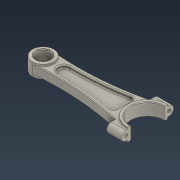
# Autodesk Inventor part: Korbowód
Saved by Autodesk Inventor 2022 (Build 260153000, 153)
## iProperties
Created: 2023-05-22
Part Number: Korbowód
Material: Generic
Document SubType Name: Modeling
Designer: wikto
Density: 1 g/cm^3
Appearance: Steel - Cast
Author: wikto
Autodesk Inventor part; units mm, degrees
ref_plane "YZ Plane" through (0, 0, 0) normal (1, 0, 0) x (0, 1, 0)
ref_plane "XZ Plane" through (0, 0, 0) normal (0, 1, 0) x (-1, 0, 0)
ref_plane "XY Plane" through (0, 0, 0) normal (0, 0, 1) x (1, 0, 0)
sketch "Sketch1" plane through (0, 0, 0) normal (0, 1, 0) x (-1, 0, 0)
  circle A0 centre (49, 0) radius 11
  arc A1 (-121, -27.5) -> (-121, 27.5) centre (-121, 0) ccw
  circle A2 centre (49, 0) radius 12.5
  circle A3 centre (49, 0) radius 17.5
  arc A4 (-121, -32.5) -> (-121, 32.5) centre (-121, 0) ccw
  line L0 (-121, -32.5) -> (-121, -42.5)
  line L1 (-121, -42.5) -> (-96, -42.5)
  line L2 (-121, 32.5) -> (-121, 42.5)
  line L3 (-121, 42.5) -> (-96, 42.5)
  line L4 (-96, -42.5) -> (-96, -27.5)
  line L5 (-96, 42.5) -> (-96, 27.5)
  arc A5 (49, -17.5) -> (-96, -27.5) centre (7.0545, -465.5408) ccw
  arc A6 (-96, 27.5) -> (49, 17.5) centre (7.0545, 465.5408) ccw
  line L6 (-121, -32.5) -> (-121, -27.5)
  line L7 (-121, 32.5) -> (-121, 27.5)
  point P0 (0, 0)
  point P1 (45.8719, 17.2182)
  point P2 (45.8719, -17.2182)
  dimension "d0" = 170
  dimension "d1" = 22
  dimension "d2" = 55
  dimension "d3" = 121
  dimension "d4" = 25
  dimension "d5" = 35
  dimension "d7" = 65
  dimension "d8" = 25
  dimension "d9" = 10
  dimension "d10" = 15
  dimension "d11" = 450
  constraints: 16 end point, 10 point on circle, 7 centre point, 6 vertical, 6 vertical alignment, 3 coincident, 3 equal length, 2 horizontal alignment, 2 perpendicular, 2 point on line, 1 equal radius
  measures "d0" distance of A1.centre A0.centre
  measures "d1" diameter of A0
  measures "d2" diameter of A1
  measures "d3" distance of A1.centre point (0, 0)
  measures "d4" diameter of A2
  measures "d5" diameter of A3
  measures "d7" diameter of A4
  measures "d8" distance of L0.end L1.end
  measures "d9" distance of L0.start L0.end
  measures "d10" distance of L1.end L4.end
  measures "d11" radius of A6
extrude "Extrusion1" add sketch "Sketch1" along normal mid plane 21 contours A1 L7 A4 L6 | A3 A6 A5
extrude "Extrusion2" add sketch "Sketch1" along normal mid plane 15 contours A4 L2 L3 L5 A6 A3 A5 L4 L1 L0
extrude "Extrusion3" add sketch "Sketch1" along normal mid plane 23 contours A2
sketch "Sketch2" plane through (0, 7.5, 0) normal (0, 1, 0) x (1, 0, 0)
  arc A0 (-45.8719, 17.2182) -> (96, 27.5) centre (-7.0545, 465.5408) ccw projected
  arc A1 (96, -27.5) -> (-45.8719, -17.2182) centre (-7.0545, -465.5408) ccw projected
  arc A2 (-14.836, 9.6072) -> (77.0775, 17.3692) centre (-7.0545, 465.5408) ccw
  arc A3 (77.0775, -17.3692) -> (-14.836, -9.6072) centre (-7.0545, -465.5408) ccw
  line L0 (83, 12.455) -> (83, -12.455)
  arc A4 (83, 12.455) -> (77.0775, 17.3692) centre (78, 12.455) ccw
  arc A5 (77.0775, -17.3692) -> (83, -12.455) centre (78, -12.455) ccw
  arc A6 (-14.836, 9.6072) -> (-14.836, -9.6072) centre (-15, 0) ccw
  point P0 (0, 0)
  point P1 (83, 0)
  dimension "d18" = 6
  dimension "d19" = 15
  dimension "d20" = 83
  dimension "d21" = 5
  constraints: 10 point on circle, 6 tangent, 5 centre point, 2 end point, 1 horizontal alignment, 1 midpoint, 1 vertical, 1 vertical alignment
  measures "d18" radial gap between concentric circles of A2 A0
  measures "d19" distance of point (0, 0) A6.centre
  measures "d20" distance of point (83, 0) point (0, 0)
  measures "d21" radius of A4
extrude "Extrusion4" cut sketch "Sketch2" against normal blind 5
sketch "Sketch3" plane through (96, -7.5, -27.5) normal (-1, 0, 0) x (0, 0, 1)
  line L0 (-15, 0) -> (-15, 15) projected
  line L1 (55, 15) -> (70, 15) projected
  line L2 (-15, 15) -> (0, 15) projected
  point P0 (27.5, 7.5)
  point P1 (-7.5, 7.5)
  point P2 (62.5, 7.5)
  point P3 (-15, 7.5)
  point P4 (62.5, 15)
  point P5 (-7.5, 15)
  constraints: 3 midpoint, 2 horizontal alignment, 2 vertical alignment
hole "Hole1" at (96, 0, -35) at (96, 0, 35) direction (1, 0, 0) diameter 5 end through all
mirror "Mirror1" about plane through (0, 0, 0) normal (0, 1, 0) of "Extrusion4"
fillet "Fillet1" radius 2 26 edges at (81.1928, 7.5, -16.3029) (83, 7.5, 0) (81.1928, 7.5, 16.3029) (31.3175, 7.5, 11.1582) (-24.6086, 7.5, 0) (31.3175, 7.5, -11.1582) (81.1928, 2.5, -16.3029) (83, 2.5, 0) (81.1928, 2.5, 16.3029) (31.3175, 2.5, 11.1582) (-24.6086, 2.5, 0) (31.3175, 2.5, -11.1582) (96, 0, 27.5) (96, 0, -27.5) (-24.6086, -2.5, 0) (31.3175, -2.5, -11.1582) (81.1928, -2.5, -16.3029) (83, -2.5, 0) (81.1928, -2.5, 16.3029) (31.3175, -2.5, 11.1582) (81.1928, -7.5, 16.3029) (83, -7.5, 0) (81.1928, -7.5, -16.3029) (31.3175, -7.5, -11.1582) (-24.6086, -7.5, 0) (31.3175, -7.5, 11.1582)
full round fillet "Full Round Fillet1" first side at (110.0741, -7.5, -38.8519) centre faces at (112.6667, 2.5, 42.5) second side at (110.0741, 7.5, -38.8519)
full round fillet "Full Round Fillet2" first side at (110.0741, -7.5, -38.8519) centre faces at (112.6667, -2.5, -42.5) second side at (110.0741, 7.5, -38.8519)
chamfer "Chamfer1" distance 1 angle 45 4 edges at (93.5, 10.5, 0) (93.5, -10.5, 0) (-38, 11.5, 0) (-38, -11.5, 0)
fillet "Fillet3" radius 1 2 edges at (88.5, 7.5, 0) (88.5, -7.5, 0)
chamfer "Chamfer2" distance 1 angle 45 16 edges at (96, 5.3033, 40.3033) (96, -5.3033, 40.3033) (96, -7.5, 32.0435) (95.5656, -7.5, 27.8424) (24.6797, -7.5, 16.6612) (96, 7.5, 32.0435) (95.5656, 7.5, 27.8424) (24.6797, 7.5, 16.6612) (24.6797, 7.5, -16.6612) (95.5656, 7.5, -27.8424) (96, 7.5, -32.0435) (96, 5.3033, -40.3033) (96, -5.3033, -40.3033) (96, -7.5, -32.0435) (95.5656, -7.5, -27.8424) (24.6797, -7.5, -16.6612)
body "Solid1"
